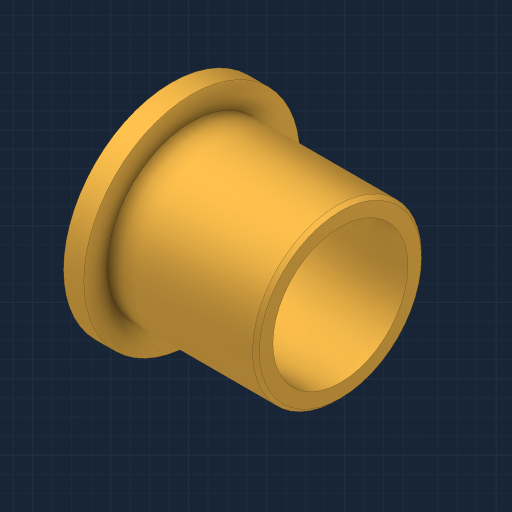
# Autodesk Inventor part: 03-bushing
Saved by Autodesk Inventor 2024 (Build 280153000, 153)
## iProperties
Created: 2025-03-09
Part Number: 03-bushing
Material: Brass, Soft Yellow
Document SubType Name: Modeling
Designer: DuctopwH
Density: 8.47 g/cm^3
Appearance: Brass - Satin
Author: DuctopwH
Autodesk Inventor part; units mm, degrees
ref_plane "YZ Plane" through (0, 0, 0) normal (1, 0, 0) x (0, 1, 0)
ref_plane "XZ Plane" through (0, 0, 0) normal (0, 1, 0) x (-1, 0, 0)
ref_plane "XY Plane" through (0, 0, 0) normal (0, 0, 1) x (1, 0, 0)
sketch "Sketch1" plane through (0, 0, 0) normal (0, 0, 1) x (1, 0, 0)
  line L0 (-12.5, 0) -> (0, 0)
  line L1 (0, 0) -> (12.5, 0)
  line L2 (-12.5, 10) -> (-12.5, 16)
  line L3 (-12.5, 16) -> (-9.5, 16)
  line L4 (-9.5, 16) -> (-9.5, 12.5)
  line L5 (-9.5, 12.5) -> (12.5, 12.5)
  line L6 (12.5, 12.5) -> (12.5, 10)
  line L7 (12.5, 10) -> (-12.5, 10)
  dimension "d0" = 25
  dimension "d1" = 22
  dimension "d2" = 20
  dimension "d3" = 25
  dimension "d4" = 32
  constraints: 17 end point, 5 perpendicular, 3 point on line, 1 collinear, 1 horizontal, 1 vertical
  measures "d0" distance between parallel lines of L6 L2
  measures "d1" distance between parallel lines of L6 L4
  measures "d2" diameter of L7 L1
  measures "d3" diameter of L5 L1
  measures "d4" diameter of L3 L0
revolve "Revolution1" add sketch "Sketch1" angle 360 about axis through (-12.5, 0, 0) along (1, 0, 0)
chamfer "Chamfer1" distance 0.5 angle 45 1 edges at (12.5, -12.5, 0)
body "Solid1"
